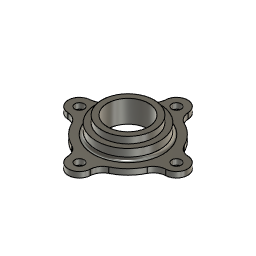
TóthMártonMarcell_hazi2 (Autodesk Fusion 360 design; units mm, degrees)
Autodesk Fusion 360 part; units mm, degrees
note: some values were not read from the file. Set by a fixed rule: which sketch regions a step uses.
sketch "Sketch1" plane through (0, 0, 0) normal (0, 0, 1) x (1, 0, 0)
  circle A0 centre (0, 0) radius 26
  circle A1 centre (0, 0) radius 17
  circle A2 centre (0, 0) radius 14
  circle A3 centre (0, 0) radius 11
  circle A4 centre (-26, 0) radius 2.5
  line L0 (1.75, 0) -> (22.5, 0)
  arc A5 (-22.0433, 4.5105) -> (-22.0433, -4.5105) centre (0, 0) ccw
  arc A6 (22.5, 0) -> (-20.2009, 9.9083) centre (0, 0) ccw
  arc A7 (-20.2009, -9.9083) -> (22.5, 0) centre (0, 0) ccw
  arc A8 (-26.2241, 5.9958) -> (-26.2241, -5.9958) centre (-26, 0) ccw
  arc A9 (-22.0433, -4.5105) -> (-22.0433, 4.5105) centre (-26, 0) ccw
  arc A10 (-26.2241, 5.9958) -> (-20.2009, 9.9083) centre (-26.4856, 12.9909) ccw
  arc A11 (-20.2009, -9.9083) -> (-26.2241, -5.9958) centre (-26.4856, -12.9909) ccw
  arc A12 (-5.9958, -26.2241) -> (5.9958, -26.2241) centre (0, -26) ccw
  circle A13 centre (0, -26) radius 2.5
  arc A14 (-5.9958, -26.2241) -> (-9.9083, -20.2009) centre (-12.9909, -26.4856) ccw
  arc A15 (9.9083, -20.2009) -> (5.9958, -26.2241) centre (12.9909, -26.4856) ccw
  arc A16 (26.2241, -5.9958) -> (26.2241, 5.9958) centre (26, 0) ccw
  circle A17 centre (26, 0) radius 2.5
  arc A18 (26.2241, -5.9958) -> (20.2009, -9.9083) centre (26.4856, -12.9909) ccw
  arc A19 (20.2009, 9.9083) -> (26.2241, 5.9958) centre (26.4856, 12.9909) ccw
  arc A20 (5.9958, 26.2241) -> (-5.9958, 26.2241) centre (0, 26) ccw
  circle A21 centre (0, 26) radius 2.5
  arc A22 (5.9958, 26.2241) -> (9.9083, 20.2009) centre (12.9909, 26.4856) ccw
  arc A23 (-9.9083, 20.2009) -> (-5.9958, 26.2241) centre (-12.9909, 26.4856) ccw
  dimension "d6" = 26
  dimension "d7" = 22.5
  dimension "d8" = 14
  dimension "d9" = 11
  dimension "d10" = 17
  dimension "d12" = 6
  dimension "d14" = 2.5
  dimension "d15" = 7
  dimension "d16" = 7
  dimension "d18" = 360
  constraint coincident A0.centre A1.centre
  constraint concentric A0 A5
  constraint concentric A0 A2
  constraint concentric A0 A3
  constraint concentric A0 A1
  constraint concentric A4 A8
  constraint coincident A4.centre L0
  constraint coincident A0 A4.centre
  constraint concentric A5 A6
  constraint concentric A5 A7
  constraint concentric A8 A9
  constraint tangent A6 A10
  constraint tangent A8 A10
  constraint coincident A5.end A8
  constraint tangent A7 A11
  constraint tangent A8 A11
  measures "d6" radius of A0
  measures "d7" radius of A5
  measures "d8" radius of A2
  measures "d9" radius of A3
  measures "d10" radius of A1
  measures "d12" radius of A8
  measures "d14" radius of A4
  measures "d15" radius of A10
  measures "d16" radius of A11
extrude "Extrude3" add sketch "Sketch1" along normal blind 3 contours A0 A6 A7 A17 A18 A19 | A0 A16 A17 A18 A19 | A0 A6 A21 A22 A23 | A0 A20 A21 A22 A23 | A0 A4 A6 A7 A10 A11 | A0 A12 A13 A14 A15 | A0 A7 A13 A14 A15 | A0 A4 A8 A10 A11 | A5 A9
extrude "Extrude4" add sketch "Sketch1" along normal blind 8.5 contours A1
extrude "Extrude5" add sketch "Sketch1" along normal blind 12 contours A2
fillet "Fillet1" radius 1.5 1 edges at (-15.8496, 6.1475, 3)
equation "d27 = 3 mm + 5.5 mm + 3.5 mm"
